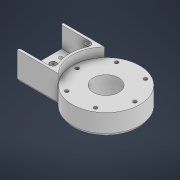
# Autodesk Inventor part: Fixed_Link_Fixation_Large
Saved by Autodesk Inventor 2021 (Build 250183000, 183)
## iProperties
Created: 2025-04-02
Part Number: Fixed_Link_Fixation_Large
Material: Generic
Document SubType Name: Modeling
Designer: rocke
Density: 1 g/cm^3
Appearance: Default
3D_PRINTED: True
Author: rocke
Autodesk Inventor part; units mm, degrees
ref_plane "YZ Plane" through (0, 0, 0) normal (1, 0, 0) x (0, 1, 0)
sketch "Sketch1" plane through (0, 0, 0) normal (0, 1, 0) x (-1, 0, 0)
  circle A0 centre (0, 0) radius 41
  circle A1 centre (0, 0) radius 37
  dimension "d0" = 82
  dimension "d3" = 74
  constraints: 2 centre point, 2 coincident
  measures "d0" diameter of A0
  measures "d3" diameter of A1
extrude "Extrusion1" add sketch "Sketch1" along normal blind 25 contours A0 | A1
chamfer "Chamfer1" distance 3 distance2 2 1 edges at (41, 0, 0) measured on face at (41, 0.5, 0)
ref_plane "Work Plane5" through (0, 11.1, 0) normal (0, -1, 0) x (1, 0, 0)
sketch "Sketch4" plane through (0, 11.1, 0) normal (0, 1, 0) x (1, 0, 0)
  line L0 (0, 28.1) -> (-80, 28.1)
  line L1 (-80, 28.1) -> (-80, -28.1)
  line L2 (-80, -28.1) -> (0, -28.1)
  line L3 (0, -28.1) -> (0, 28.1)
  line L4 (0, 0) -> (-41, 0)
  circle A0 centre (0, 0) radius 41 projected
  line L5 (-77, -25.1) -> (-77, 25.1)
  line L6 (-77, 25.1) -> (-3, 25.1)
  line L7 (-3, 25.1) -> (-3, -25.1)
  line L8 (-3, -25.1) -> (-77, -25.1)
  line L9 (-77, 25.1) -> (-80, 25.1)
  line L10 (-77, -25.1) -> (-80, -25.1)
  point P0 (-29.8562, -28.1)
  point P1 (-32.419, -25.1)
  point P2 (-32.419, 25.1)
  point P3 (-29.8562, 28.1)
  dimension "d22" = 56.2
  dimension "d23" = 80
  dimension "d24" = 3
  constraints: 22 end point, 4 parallel, 4 perpendicular, 2 horizontal, 2 point on line, 1 midpoint, 6 other
  measures "d22" distance of L2.end L0.start
  measures "d23" distance between parallel lines of L3 L1
  measures "d24" distance between parallel lines of L1 L5
extrude "Extrusion3" add sketch "Sketch4" along normal blind 25.2 contours A0 L6 L9 L1 L0 | A0 L8 L5 L6 | L9 L5 L10 L1 | L2 L1 L10 L8 A0
extrude "Extrusion8" add sketch "Sketch4" against normal blind 8 contours L3 L4 L7 L6 A0 L0 | A0 L6 L9 L1 L0 | L3 L2 A0 L8 L7 L4 | L6 L7 L4 A0 | A0 L8 L5 L6 | L7 L8 A0 L4 | L9 L5 L10 L1 | L2 L1 L10 L8 A0
ref_plane "Work Plane3" through (18.0218, -5.4407, 0) normal (0, 0, 1) x (1, 0, 0)
ref_plane "Work Plane4" through (0, -17.1, 0) normal (0, 1, 0) x (1, 0, 0)
sketch "Sketch13" plane through (0, 11.1, 0) normal (0, 1, 0) x (1, 0, 0)
  line L0 (-70, -25.1) -> (-70, 25.1) projected
  point P0 (0, 0)
  point P1 (-60, 30)
  dimension "d56" = 30
  dimension "d57" = 10
  measures "d56" vertical distance of point (0, 0) point (-60, 30)
  measures "d57" distance from line of L0 point (-60, 30)
sketch "Sketch14" plane through (0, 36.3, 0) normal (0, 1, 0) x (1, 0, 0)
  line L0 (-57.3383, 10.95) -> (-59.6765, 15)
  line L1 (-59.6765, 15) -> (-57.3383, 19.05)
  line L2 (-57.3383, 19.05) -> (-52.6617, 19.05)
  line L3 (-52.6617, 19.05) -> (-50.3235, 15)
  line L4 (-50.3235, 15) -> (-52.6617, 10.95)
  line L5 (-52.6617, 10.95) -> (-57.3383, 10.95)
  line L6 (-80, 28.1) -> (-80, -28.1) projected
  line L7 (-70, 25.1) -> (-70, -25.1) projected
  line L8 (-70, 0) -> (0, 0)
  line L9 (-57.3383, -10.95) -> (-59.6765, -15)
  line L10 (-59.6765, -15) -> (-57.3383, -19.05)
  line L11 (-57.3383, -19.05) -> (-52.6617, -19.05)
  line L12 (-52.6617, -19.05) -> (-50.3235, -15)
  line L13 (-50.3235, -15) -> (-52.6617, -10.95)
  line L14 (-52.6617, -10.95) -> (-57.3383, -10.95)
  line L15 (-67.6617, 10.95) -> (-72.3383, 10.95)
  line L16 (-72.3383, 10.95) -> (-74.6765, 15)
  line L17 (-65.3235, 15) -> (-67.6617, 10.95)
  line L18 (-74.6765, 15) -> (-72.3383, 19.05)
  line L19 (-72.3383, 19.05) -> (-67.6617, 19.05)
  line L20 (-67.6617, 19.05) -> (-65.3235, 15)
  line L21 (-67.6617, -10.95) -> (-72.3383, -10.95)
  line L22 (-72.3383, -10.95) -> (-74.6765, -15)
  line L23 (-65.3235, -15) -> (-67.6617, -10.95)
  line L24 (-67.6617, -19.05) -> (-65.3235, -15)
  line L25 (-72.3383, -19.05) -> (-67.6617, -19.05)
  line L26 (-74.6765, -15) -> (-72.3383, -19.05)
  point P0 (-55, 15)
  point P1 (-80, -28.1)
  point P2 (-55, -15)
  point P3 (-70, 15)
  point P4 (-70, -15)
  dimension "d58" = 8.1
  dimension "d59" = 15
  dimension "d60" = 25
  dimension "d63" = 15
  constraints: 50 end point, 7 symmetric about line, 3 horizontal, 1 midpoint, 40 other
  measures "d58" distance between parallel lines of L5 L2
  measures "d59" vertical distance of L8.end point (-55, 15)
  measures "d63" distance of point (-55, 15) point (-70, 15)
extrude "Extrusion7" cut sketch "Sketch14" along normal blind 5 from surface at -33.2
hole "Hole2" at (-55, 36.3, -15) at (-55, 36.3, 15) at (-70, 36.3, 15) at (-70, 36.3, -15) direction (0, -1, 0) diameter 4.3 end through all clearance for "Socket Head Cap Screw" size "M4" standard "Ansi Metric M Profile"
sketch "Sketch3" plane through (0, 0, 0) normal (0, -1, 0) x (1, 0, 0)
  point P0 (0, 0)
  point P1 (-35, 0)
  point P2 (17.5, -30.3109)
  point P3 (17.5, 30.3109)
  dimension "d10" = 35
  dimension "d13" = 360
  constraints: 4 other
  measures "d10" distance of point (0, 0) point (-35, 0)
hole "Hole1" at (-35, 0, 0) at (17.5, 0, -30.3109) at (17.5, 0, 30.3109) direction (0, 1, 0) diameter 4.3 end through all counterbore diameter 8 counterbore depth 4 clearance for "Socket Head Cap Screw" size "M4" standard "Ansi Metric M Profile"
pattern_circular "Circular Pattern1" count 2 over 360 about axis through (0, 0, 0) along (0, 1, 0) of "Hole1"
extrude "Extrusion9" cut sketch "Sketch4" against normal blind 25.1 from surface at 25.2 contours A0 L8 L5 L6 | L9 L5 L10 L1
sketch "Sketch15" plane through (0, 0, 0) normal (0, -1, 0) x (1, 0, 0)
  circle A0 centre (0, 0) radius 15.5
  dimension "d94" = 31
  constraints: 1 centre point, 1 coincident
  measures "d94" diameter of A0
extrude "Extrusion10" cut sketch "Sketch15" against normal through all
sketch "Sketch16" plane through (-80, 3.1, -25.1) normal (0, 1, 0) x (1, 0, 0)
  circle A0 centre (36.8863, -4) radius 4
  arc A1 (47.581, 0) -> (47.581, -50.2) centre (80, -25.1) ccw projected
  line L0 (0, 0) -> (47.581, 0) projected
  line L1 (0, 0) -> (47.581, 0) projected
  arc A2 (43.8615, 0) -> (44.5528, -51.1671) centre (80, -25.1) ccw
  point P0 (36.8863, 0)
  point P1 (43.7865, -5.8756)
  point P2 (40.4791, -5.7583)
  point P3 (43.8615, 0)
  dimension "d97" = 8
  dimension "d123" = 3
  constraints: 2 centre point, 2 point on circle, 2 tangent, 1 coincident, 1 point on line
  measures "d97" diameter of A0
  measures "d123" radial gap between concentric circles of A2 A1
extrude "Extrusion11" add sketch "Sketch16" along normal up to surface (33.2 mm away) from surface at 0
sketch "Sketch18" plane through (-80, 11.2, 25.1) normal (0, 1, 0) x (1, 0, 0)
  line L0 (50.1438, -3) -> (0, -3) projected
  arc A0 (50.1438, 53.2) -> (50.1438, -3) centre (80, 25.1) ccw
  line L1 (50.1438, 53.2) -> (0, 53.2) projected
  arc A1 (46.1416, 53.2) -> (46.1416, -3) centre (80, 25.1) ccw
  line L2 (0, -3) -> (50.1438, -3) projected
  point P0 (46.1416, -3)
  dimension "d113" = 3
  constraints: 4 point on circle, 2 centre point, 2 coincident, 2 point on line
  measures "d113" radial gap between concentric circles of A1 A0
extrude "Extrusion13" add sketch "Sketch18" along normal up to surface (25.1 mm away)
sketch "Sketch17" plane through (0, 36.3, 0) normal (0, 1, 0) x (1, 0, 0)
  arc A0 (-43.1137, 25.1) -> (-39.5209, 19.3417) centre (-43.1137, 21.1) ccw projected
  circle A1 centre (-43.1137, 21.1) radius 3.4
  point P0 (0, 0)
  dimension "d124" = 6.8
  constraints: 1 centre point, 1 coincident
  measures "d124" diameter of A1
extrude "Extrusion12" add sketch "Sketch17" along normal blind 1
chamfer "Chamfer5" distance 0.5 angle 45 1 edges at (-46.5137, 37.3, -21.1)
hole "Hole4" at (-43.1137, 3.1, -21.1) direction (0, 1, 0) diameter 4.3 end through all counterbore diameter 8 counterbore depth 4 clearance for "Socket Head Cap Screw" size "M4" standard "Ansi Metric M Profile"
mirror "Mirror3" about plane through (0, 0, 0) normal (0, 0, 1) of "Extrusion11", "Extrusion12", "Chamfer5", "Hole4"
chamfer "Chamfer6" distance 1 angle 45 3 edges at (-80, 23.75, 25.1) (-80, 11.2, 0) (-80, 23.75, -25.1)
chamfer "Chamfer7" distance 2 distance2 3 1 edges at (-54.9281, 3.1, 28.1) measured on face at (-54.9281, 3.1, 27.6)
chamfer "Chamfer8" distance 2 distance2 3 1 edges at (-54.9281, 3.1, -28.1) measured on face at (-54.9281, 3.1, -27.6)
fillet "Fillet3" radius 3 2 edges at (-29.8562, 15.55, 28.1) (-29.8562, 15.55, -28.1)
equation "\"d3\" = OD - 2 * WALL_THICKNESS"
equation "\"d22\" = 2 * WALL_THICKNESS + LINK_HEIGHT + TRANSITION"
equation "\"d25\" = 0.5 * LINK_WIDTH + TRANSITION"
equation "\"WALL_THICKNESS\" = 3"
equation "\"M4_THICKNESS\" = 8"
equation "\"TRANSITION\" = 0.2"
equation "\"CHAMFER_Y\" = 3"
equation "\"OD\" = 80"
equation "\"LINK_HEIGHT\" = 50"
equation "\"LINK_WIDTH\" = 50"
body "Solid1"
